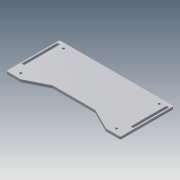
# Autodesk Inventor part: FrontPanel
Saved by Autodesk Inventor 2014 (Build 180170000, 170)
## iProperties
Created: 2015-01-19
Part Number: FrontPanel
Material: Generic
Document SubType Name: Modeling
Designer: Peele
Density: 1 g/cm^3
Appearance: White
Author: Peele
Autodesk Inventor part; units mm, degrees
ref_plane "YZ Plane" through (0, 0, 0) normal (1, 0, 0) x (0, 1, 0)
ref_plane "XZ Plane" through (0, 0, 0) normal (0, 1, 0) x (-1, 0, 0)
ref_plane "XY Plane" through (0, 0, 0) normal (0, 0, 1) x (1, 0, 0)
sketch "Sketch1" plane through (0, 0, 0) normal (0, 0, 1) x (1, 0, 0)
  line L0 (0, 0) -> (0, 125)
  line L1 (0, 125) -> (268, 125)
  line L2 (268, 125) -> (268, 0)
  line L3 (268, 0) -> (0, 0)
  point P0 (134, 125)
  dimension "d1" = 125
  dimension "d2" = 268
  constraints: 8 end point, 2 horizontal, 2 vertical, 1 midpoint
  measures "d1" distance of L1.end L2.end
  measures "d2" distance of L2.end L0.start
extrude "Extrusion1" add sketch "Sketch1" along normal blind 6
sketch "Sketch2" plane through (0, 0, 6) normal (0, 0, 1) x (1, 0, 0)
  line L0 (0, 0) -> (268, 0) projected
  line L1 (268, 0) -> (268, 125) projected
  line L2 (34, 0) -> (84, 25)
  line L3 (84, 25) -> (184, 25)
  line L4 (184, 25) -> (234, 0)
  line L5 (234, 0) -> (34, 0)
  line L6 (0, 125) -> (0, 0) projected
  dimension "d6" = 25
  dimension "d7" = 34
  dimension "d9" = 50
  dimension "d47" = 34
  constraints: 8 end point, 2 point on line, 1 collinear, 1 equal length, 1 parallel
  measures "d6" distance between parallel lines of L0 L3
  measures "d7" distance from line of L4.end L1
  measures "d9" horizontal distance of L2.end L2.start
  measures "d47" distance from line of L6 L2.start
extrude "Extrusion2" cut sketch "Sketch2" against normal through all
sketch "Sketch7" plane through (0, 0, 6) normal (0, 0, 1) x (1, 0, 0)
  line L0 (268, 0) -> (268, 125) projected
  line L1 (268, 125) -> (0, 125) projected
  line L2 (0, 125) -> (0, 0) projected
  line L3 (0, 0) -> (34, 0) projected
  line L4 (84, 25) -> (184, 25) projected
  circle A0 centre (246.5, 12.5) radius 2.7
  circle A1 centre (246.5, 112.5) radius 2.7
  circle A2 centre (21.5, 12.5) radius 2.7
  circle A3 centre (21.5, 112.5) radius 2.7
  line L5 (2.875, 33) -> (9.125, 33)
  line L6 (9.125, 33) -> (9.125, 117)
  line L7 (9.125, 117) -> (2.875, 117)
  line L8 (2.875, 117) -> (2.875, 33)
  line L9 (2.875, 33) -> (9.125, 117) construction
  line L10 (9.125, 33) -> (2.875, 117) construction
  line L11 (258.875, 33) -> (265.125, 33)
  line L12 (265.125, 33) -> (265.125, 117)
  line L13 (265.125, 117) -> (258.875, 117)
  line L14 (258.875, 117) -> (258.875, 33)
  line L15 (258.875, 33) -> (265.125, 117) construction
  line L16 (265.125, 33) -> (258.875, 117) construction
  point P0 (6, 75)
  point P1 (262, 75)
  point P2 (6, 75)
  point P3 (262, 75)
  dimension "d48" = 21.5
  dimension "d49" = 21.5
  dimension "d50" = 12.5
  dimension "d51" = 12.5
  dimension "d56" = 2.875
  dimension "d57" = 6.25
  dimension "d58" = 2.875
  dimension "d59" = 8
  dimension "d60" = 8
  dimension "d61" = 5.4
  dimension "d62" = 84
  constraints: 24 end point, 6 midpoint, 4 centre point, 4 parallel, 3 equal radius, 3 horizontal alignment, 2 equal length, 2 horizontal, 2 perpendicular, 2 vertical alignment
  measures "d48" distance from line of A3.centre L2
  measures "d49" distance from line of A1.centre L0
  measures "d50" distance from line of A3.centre L1
  measures "d51" distance from line of A2.centre L3
  measures "d56" distance between parallel lines of L2 L8
  measures "d57" distance of L6.end L7.end
  measures "d58" distance between parallel lines of L12 L0
  measures "d59" distance between parallel lines of L5 L4
  measures "d60" distance between parallel lines of L1 L7
  measures "d61" diameter of A3
  measures "d62" distance of L5.end L6.end
extrude "Extrusion5" cut sketch "Sketch7" against normal through all
fillet "Fillet1" radius 2 8 edges at (268, 125, 3) (268, 0, 3) (234, 0, 3) (184, 25, 3) (84, 25, 3) (34, 0, 3) (0, 0, 3) (0, 125, 3)
equation "\"d7\" = d47"
equation "\"d49\" = d48"
equation "\"d51\" = d50"
equation "\"d58\" = d56"
body "Solid1"
